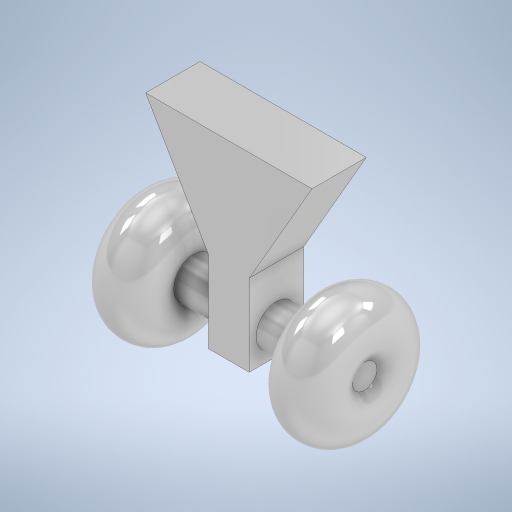
# Autodesk Inventor part: wheels
Saved by Autodesk Inventor 2024 (Build 280153000, 153)
## iProperties
Created: 2023-07-07
Part Number: wheels
Material: Generic
Document SubType Name: Modeling
Designer: tamiz
Density: 1 g/cm^3
Appearance: Default
Author: tamiz
Autodesk Inventor part; units mm, degrees
ref_plane "YZ Plane" through (0, 0, 0) normal (1, 0, 0) x (0, 1, 0)
ref_plane "XZ Plane" through (0, 0, 0) normal (0, 1, 0) x (-1, 0, 0)
ref_plane "XY Plane" through (0, 0, 0) normal (0, 0, 1) x (1, 0, 0)
sketch "Sketch1" plane through (0, 0, 0) normal (0, 0, 1) x (1, 0, 0)
  line L0 (457.2, 1219.2) -> (457.2, -609.6)
  line L1 (-457.2, -609.6) -> (-457.2, 1219.2)
  line L2 (-457.2, 1219.2) -> (-1865.0109, 3657.6)
  line L3 (457.2, 1219.2) -> (1865.0109, 3657.6)
  line L4 (-1865.0109, 3657.6) -> (1865.0109, 3657.6)
  line L5 (457.2, -609.6) -> (-457.2, -609.6)
  constraints: 12 end point, 1 horizontal, 1 perpendicular
extrude "Extrusion1" add sketch "Sketch1" along normal mid plane 1219.2
sketch "Sketch2" plane through (0, 0, 0) normal (1, 0, 0) x (0, 1, 0)
  circle A0 centre (0, 0) radius 457.2
  constraints: 1 centre point, 1 coincident
extrude "Extrusion2" add sketch "Sketch2" along normal mid plane 4876.8
sketch "Sketch3" plane through (0, 0, 0) normal (0, 0, 1) x (1, 0, 0)
  line L0 (-2919.5032, 0) -> (3069.2275, 0) construction
  line L1 (2438.4, -457.2) -> (2438.4, 457.2) projected
  line L2 (457.2, 457.2) -> (2438.4, 457.2) projected
  circle A0 centre (1981.2, 762) radius 665.6271
  point P0 (2438.4, 278.236)
  point P1 (1389.4599, 457.2)
  constraints: 2 end point, 1 centre point, 1 horizontal
revolve "Revolution1" add sketch "Sketch3" angle 360 about axis through (-2919.5032, 0, 0) along (1, 0, 0) picked at (1765.7699, 908.3284) contours L1 L2 A0
mirror "Mirror1" about plane through (0, 0, 0) normal (1, 0, 0) of "Revolution1"
body "Solid1"
